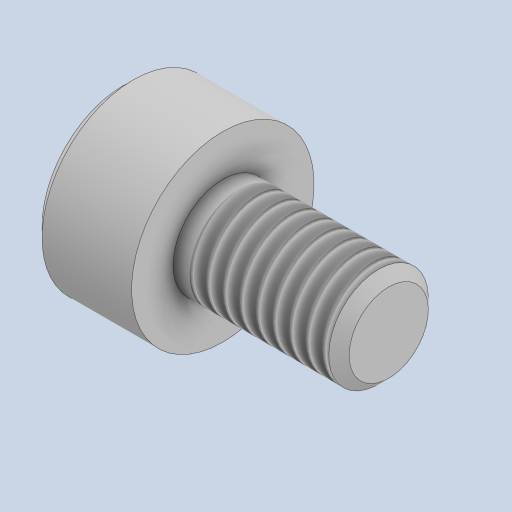
# Autodesk Inventor part: CBE3-5
Saved by Autodesk Inventor 2023 (Build 270158000, 158)
## iProperties
Category: PARTsolutions
Company: MISUMI
Created: 2024-12-10
Part Number: CBE3-5
Material: Generic
Catalog Web Link: www.cadenas.de
Description: CBE-Hexagon Socket Head Cap Screws -Trivalent Chromate-
Vendor: MISUMI
Document SubType Name: Modeling
Designer: psAdmin
Manufacturer: MISUMI
Mass: 0.0972387 g
Surface Area: 1.53526 cm^2
Volume: 0.0972387 cm^3
Density: 1 g/cm^3
Appearance: PSOLRGB-175-175-175
PSOL_IDENT_0: {$CADENAS_DATA/23d-libs/misumi/metric/27_screws_nuts/cbe.prj},151 {VTYP=3D},{NB=CBE3-5},{LINA=CBE3-5
PSOL_IDENT_1: },{NN=CBE},{DATE=29.11.2024 04:24:12},{GEOMDATE=29.01.2020 09:52:26},{VERSION=},{LINEID=40},{WBVAR=L
PSOL_IDENT_2: },{WBNUMERIC=L}  {NB=CBE3-5},{LINA=CBE3-5},{KT=DUMMY},{PN=CBE3-5},{TYPE=CBE},{M=3},{M1=3.0},{L=5},{L
PSOL_IDENT_3: 0=4,5,6,8,10,12,15,18,20,25,30,35},{LL1=5},{LL=Full Thread},{P=0.50},{A=5.5},{E=3.0},{B=2.5},{TT=1.3
PSOL_IDENT_4: },{VV=0.30}
NB: CBE3-5
NN: CBE
NT: Hexagon Socket Head Cap Screws -Trivalent Chromate-
NBSYN: $PN.
LINA: CBE3-5
CATALOG: Misumi
PN: CBE3-5
M: 3
L: 5
LL: Full Thread
P: 0.5
A: 5.5
E: 3
B: 2.5
SUPPLIER: MISUMI
ARTICLENO: CBE3-5
BOMINFO: CBE3-5
CREATOR: CADENAS GmbH
Title: CBE3-5
Author: Cadenas PARTsolutions
Comments: Hexagon Socket Head Cap Screws -Trivalent Chromate-
Autodesk Inventor part; units mm, degrees
sketch "Sketch_1" plane through (0, 0, 0) normal (0, 0, 1) x (1, 0, 0)
  line L0 (5, 0) -> (-3, 0)
  line L1 (-3, 0) -> (-3, 2.45)
  line L2 (-3, 2.45) -> (-2.7, 2.75)
  line L3 (-2.7, 2.75) -> (0, 2.75)
  line L4 (0, 2.75) -> (0, 1.5)
  line L5 (0, 1.5) -> (4.6935, 1.5)
  line L6 (4.6935, 1.5) -> (5, 1.1935)
  line L7 (5, 1.1935) -> (5, 0)
  line L8 (5, 0) -> (-3, 0)
  constraints: 18 end point
revolve "Revolution1" add sketch "Sketch_1" angle 360 about axis through (5, 0, 0) along (1, 0, 0)
thread "Thread1" size "M3x0.5" class "6g" standard "ISO Metric profile" length 4.1935
sketch "Sketch2" plane through (-3, 0, 0) normal (-1, 0, 0) x (0, 0, 1)
  point P0 (0, 0)
hole "Hole1" at (-3, 0, 0) direction (1, 0, 0) diameter 2.5 depth 1.3 tip angle 120
sketch "Sketch_3" plane through (-3, 0, 0) normal (1, 0, 0) x (0, 0, -1)
  line L0 (-1.25, -0.7217) -> (0, -1.4434)
  line L1 (0, -1.4434) -> (1.25, -0.7217)
  line L2 (1.25, -0.7217) -> (1.25, 0.7217)
  line L3 (1.25, 0.7217) -> (0, 1.4434)
  line L4 (0, 1.4434) -> (-1.25, 0.7217)
  line L5 (-1.25, 0.7217) -> (-1.25, -0.7217)
  constraints: 12 end point
extrude "Extrusion1" cut sketch "Sketch_3" along normal blind 1.3
ref_plane "bolt_XY" through (5, 0, 0) normal (1, 0, 0) x (0, 0, -1)
ref_plane "bolt_YZ" through (5, 0, 0) normal (0, 0, -1) x (0, 1, 0)
ref_plane "bolt_ZX" through (5, 0, 0) normal (0, 1, 0) x (1, 0, 0)
ref_plane "nut_XY" through (0, 0, 0) normal (1, 0, 0) x (0, 0, -1)
ref_plane "nut_YZ" through (0, 0, 0) normal (0, 0, -1) x (0, 1, 0)
ref_plane "nut_ZX" through (0, 0, 0) normal (0, 1, 0) x (1, 0, 0)
body "Solid1"
